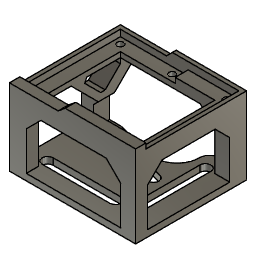
header_bus_mount v4 (Autodesk Fusion 360 design; units mm, degrees)
Autodesk Fusion 360 part; units mm, degrees
sketch "Sketch1" plane through (0, 0, 0) normal (0, 0, 1) x (1, 0, 0)
  line L0 (17.22, 32.84) -> (37.54, 32.84) construction
  line L1 (37.54, 32.84) -> (37.54, 1.4) construction
  line L2 (37.54, 1.4) -> (17.22, 1.4) construction
  line L3 (17.22, 1.4) -> (17.22, 32.84) construction
  line L4 (1.4, 32.84) -> (21.72, 32.84) construction
  line L5 (21.72, 32.84) -> (21.72, 1.4) construction
  line L6 (21.72, 1.4) -> (1.4, 1.4) construction
  line L7 (1.4, 1.4) -> (1.4, 32.84) construction
  line L8 (1.2, 33.04) -> (37.74, 33.04)
  line L9 (37.74, 33.04) -> (37.74, 1.2)
  line L10 (37.74, 1.2) -> (1.2, 1.2)
  line L11 (1.2, 1.2) -> (1.2, 33.04)
  line L12 (38.94, 34.24) -> (38.94, 0)
  line L13 (38.94, 0) -> (0, 0)
  line L14 (0, 0) -> (0, 34.24)
  line L15 (0, 34.24) -> (38.94, 34.24)
  dimension "d5" = 20.32
  dimension "d6" = 31.44
  dimension "d7" = 4.5
  dimension "d14" = 0.2
  dimension "d15" = 0.2
  dimension "d16" = 0.2
  dimension "d17" = 0.2
  constraint horizontal L0
  constraint vertical L1
  constraint horizontal L2
  constraint vertical L3
  constraint horizontal L4
  constraint vertical L5
  constraint horizontal L6
  constraint vertical L7
  constraint coincident L2 L5.end
  constraint equal L0 L4
  constraint equal L1 L7
  constraint horizontal L8
  constraint vertical L9
  constraint horizontal L10
  constraint vertical L11
  constraint coincident L13.end L14.start
  measures "d5" distance of L0.start L0.end
  measures "d6" distance of L0.end L1.end
  measures "d7" distance of L3 L5
  measures "d14" distance of L4 L8
  measures "d15" distance of L6 L10
  measures "d16" distance of L7 L11
  measures "d17" distance of L1 L9
extrude "Extrude1" add sketch "Sketch1" along normal blind 2 makes body 1
sketch "Sketch2" plane through (0, 0, 0) normal (0, 0, -1) x (1, 0, 0)
  line L0 (1.2, -1.2) -> (37.74, -1.2)
  line L1 (37.74, -1.2) -> (37.74, -33.04)
  line L2 (37.74, -33.04) -> (1.2, -33.04)
  line L3 (1.2, -33.04) -> (1.2, -1.2)
  line L4 (0, 0) -> (0, -34.24)
  line L5 (0, -34.24) -> (38.94, -34.24)
  line L6 (38.94, -34.24) -> (38.94, 0)
  line L7 (38.94, 0) -> (0, 0)
  line L8 (5.2, -3.7) -> (34.34, -3.7)
  line L9 (34.34, -3.7) -> (34.34, -29.04)
  line L10 (34.34, -29.04) -> (5.2, -29.04)
  line L11 (5.2, -29.04) -> (5.2, -3.7)
  dimension "d21" = 4
  dimension "d22" = 3.4
  dimension "d23" = 4
  dimension "d24" = 2.5
  constraint horizontal L8
  constraint vertical L9
  constraint horizontal L10
  constraint vertical L11
  measures "d21" distance of L2 L10
  measures "d22" distance of L1 L9
  measures "d23" distance of L3 L11
  measures "d24" distance of L0 L8
extrude "Extrude2" add sketch "Sketch2" along normal blind 1.6 contours L0 L1 L2 L3 | L4 L5 L6 L7 bodies 1
sketch "Sketch3" plane through (0, 0, 2) normal (0, 0, 1) x (-1, 0, 0)
  line L0 (-37.74, -1.2) -> (-1.2, -1.2)
  line L1 (-1.2, -1.2) -> (-1.2, -33.04)
  line L2 (-1.2, -33.04) -> (-37.74, -33.04)
  line L3 (-37.74, -33.04) -> (-37.74, -1.2)
  line L4 (0, -34.24) -> (0, 0)
  line L5 (0, 0) -> (-38.94, 0)
  line L6 (-38.94, 0) -> (-38.94, -34.24)
  line L7 (-38.94, -34.24) -> (0, -34.24)
  line L8 (-17.22, -1.4) -> (-17.22, -32.84) construction
  line L9 (-17.22, -34.24) -> (-17.22, -33.04)
  line L10 (-17.22, -1.2) -> (-17.22, 0)
  constraint coincident L7 L9.start
  constraint coincident L2 L9.end
  constraint perpendicular L2 L9
  constraint coincident L0 L10.start
  constraint coincident L5 L10.end
  constraint perpendicular L5 L10
  constraint collinear L8 L10
  constraint collinear L8 L9
extrude "Extrude3" add sketch "Sketch3" along normal blind 1.8 contours L0 L2 L3 L5 L6 L7 L9 L10 bodies 1
sketch "Sketch4" plane through (0, 0, 0) normal (0, 0, 1) x (-1, 0, 0)
  line L0 (-5.2, -29.04) -> (-34.34, -29.04)
  line L1 (-34.34, -29.04) -> (-34.34, -3.7)
  line L2 (-34.34, -3.7) -> (-5.2, -3.7)
  line L3 (-5.2, -3.7) -> (-5.2, -29.04)
  line L4 (-37.74, -1.2) -> (-37.74, -33.04)
  line L5 (-37.74, -33.04) -> (-1.2, -33.04)
  line L6 (-1.2, -33.04) -> (-1.2, -1.2)
  line L7 (-1.2, -1.2) -> (-37.74, -1.2)
  line L8 (-21.72, -32.84) -> (-21.72, -1.4) construction
  line L9 (-22.12, -1.2) -> (-22.12, -33.04)
  dimension "d29" = 0.4
  constraint coincident L7 L9.start
  constraint coincident L5 L9.end
  constraint perpendicular L5 L9
  measures "d29" distance of L8 L9
extrude "Extrude4" add sketch "Sketch4" along normal blind 1.6 contours L0 L1 L2 L4 L5 L7 L9 bodies 1
sketch "Sketch5" plane through (0, 0, 0) normal (0, 0, 1) x (-1, 0, 0)
  line L0 (-22.12, -29.04) -> (-22.12, -33.04)
  line L1 (-22.12, -33.04) -> (-1.2, -33.04)
  line L2 (-1.2, -33.04) -> (-1.2, -1.2)
  line L3 (-1.2, -1.2) -> (-22.12, -1.2)
  line L4 (-22.12, -1.2) -> (-22.12, -3.7)
  line L5 (-22.12, -3.7) -> (-5.2, -3.7)
  line L6 (-5.2, -3.7) -> (-5.2, -29.04)
  line L7 (-5.2, -29.04) -> (-22.12, -29.04)
  circle A0 centre (-3.2, -31.04) radius 1
  circle A1 centre (-19.2, -31.04) radius 1
  circle A2 centre (-35.94, -31.04) radius 1
  line L8 (-1.2, -1.2) -> (-1.2, -33.04)
  line L9 (-1.2, -33.04) -> (-17.22, -33.04)
  line L10 (-37.74, -33.04) -> (-37.74, -1.2) construction
  dimension "d33" = 2
  dimension "d34" = 2
  dimension "d35" = 1.8
  dimension "d36" = 18
  dimension "d37" = 2
  constraint horizontal A0.centre A1.centre
  constraint horizontal A1.centre A2.centre
  constraint equal A0 A1
  constraint equal A1 A2
  measures "d33" distance of A0.centre L8
  measures "d34" distance of A0.centre L9
  measures "d35" distance of A2.centre L10
  measures "d36" distance of A1.centre L8
  measures "d37" diameter of A0
extrude "Extrude5" cut sketch "Sketch5" along normal up to surface (-1.6 mm away) and the other way up to surface (-1.6 mm away) contours A0 | A1 | A2 bodies 1
sketch "Sketch6" plane through (0, 0, 2) normal (0, 0, 1) x (-1, 0, 0)
  line L0 (-17.22, -33.04) -> (-17.22, -34.24)
  line L1 (-17.22, -34.24) -> (0, -34.24)
  line L2 (0, -34.24) -> (0, 0)
  line L3 (0, 0) -> (-17.22, 0)
  line L4 (-17.22, 0) -> (-17.22, -1.2)
  line L5 (-17.22, -1.2) -> (-1.2, -1.2)
  line L6 (-1.2, -1.2) -> (-1.2, -33.04)
  line L7 (-1.2, -33.04) -> (-17.22, -33.04)
  line L8 (0, 0) -> (0, -3.2)
  line L9 (0, -3.2) -> (-17.02, -3.2)
  line L10 (-17.02, -3.2) -> (-17.02, 0)
  line L11 (0, 0) -> (-17.02, 0)
  line L12 (-17.22, -1.2) -> (-17.22, 0)
  dimension "d47" = 0.2
  dimension "d48" = 3.2
  constraint vertical L8
  constraint horizontal L9
  constraint coincident L2 L8.end
  constraint coincident L3 L10.end
  constraint perpendicular L3 L10
  constraint perpendicular L10 L11
  measures "d47" distance of L10 L12
  measures "d48" distance of L9 L11
extrude "Extrude6" add sketch "Sketch6" along normal blind 1.6 contours L5 L6 L9 L10 | L2 L3 L5 L6 L8 L9 L10 L11 | L3 L4 L5 L10 L12 bodies 1
sketch "Sketch7" plane through (0, 0, 3.8) normal (0, 0, 1) x (-1, 0, 0)
  line L0 (-17.22, -1.2) -> (-17.22, 0)
  line L1 (-17.22, 0) -> (-38.94, 0)
  line L2 (-38.94, 0) -> (-38.94, -34.24)
  line L3 (-38.94, -34.24) -> (-17.22, -34.24)
  line L4 (-17.22, -34.24) -> (-17.22, -33.04)
  line L5 (-17.22, -33.04) -> (-37.74, -33.04)
  line L6 (-37.74, -33.04) -> (-37.74, -1.2)
  line L7 (-37.74, -1.2) -> (-17.22, -1.2)
  line L8 (-38.94, 0) -> (-17.22, 0)
  line L9 (-17.22, 0) -> (-17.22, -3.2)
  line L10 (-17.22, -3.2) -> (-38.94, -3.2)
  line L11 (-38.94, -3.2) -> (-38.94, 0)
  line L12 (-17.02, -3.2) -> (0, -3.2)
  point P0 (-17.02, -3.2)
  point P1 (0, -3.2)
  constraint horizontal L8
  constraint vertical L9
  constraint horizontal L10
  constraint vertical L11
  constraint coincident L1.end L2.start
  constraint coincident L0.end L1.start
  constraint collinear L10 L12
extrude "Extrude7" add sketch "Sketch7" along normal blind 1.6 contours L0 L1 L2 L6 L7 L8 L9 L10 L11 | L6 L7 L9 L10 bodies 1
sketch "Sketch8" plane through (0, 3.2, 0) normal (0, 1, 0) x (-1, 0, 0)
  line L0 (-37.74, 3.8) -> (-17.22, 3.8)
  line L1 (-17.22, 3.8) -> (-17.22, 5.4)
  line L2 (-17.22, 5.4) -> (-38.94, 5.4)
  line L3 (-38.94, 5.4) -> (-38.94, 3.8)
  line L4 (-38.94, 3.8) -> (-37.74, 3.8)
  line L5 (-17.22, 5.4) -> (-15.02, 3.6)
  line L6 (-15.02, 3.6) -> (-17.02, 3.6)
  line L7 (-17.02, 3.6) -> (-17.02, 3.8)
  line L8 (-17.02, 3.8) -> (-17.22, 3.8)
  line L9 (-17.22, 3.8) -> (-17.22, 5.4)
  point P0 (-17.02, 3.6)
  dimension "d49" = 2
  constraint coincident L1.end L2.start
  constraint perpendicular L1 L6
  constraint perpendicular L0 L7
  constraint coincident L0.end L1.start
  constraint perpendicular L1 L8
  constraint coincident P0 L6.end
  measures "d49" distance of L5.end P0
extrude "Extrude8" add sketch "Sketch8" against normal up to surface (3.2 mm away) contours L1 L5 L6 L7 L8 L9 bodies 1
chamfer "Chamfer1" distance 1.8 angle 45 1 edges at (17.22, 33.64, 2) on bodies 1
sketch "Sketch9" plane through (0, 0, 0) normal (0, -1, 0) x (1, 0, 0)
  line L0 (17.22, 3.8) -> (17.22, 3.6)
  line L1 (17.22, 3.6) -> (17.02, 3.6)
  line L2 (17.02, 3.6) -> (17.02, 3.8)
  line L3 (17.02, 3.8) -> (17.22, 3.8)
  line L4 (17.22, 5.4) -> (15.02, 3.6)
  line L5 (15.02, 3.6) -> (0, 3.6)
  line L6 (0, 3.6) -> (0, -1.6)
  line L7 (0, -1.6) -> (38.94, -1.6)
  line L8 (38.94, -1.6) -> (38.94, 5.4)
  line L9 (38.94, 5.4) -> (17.22, 5.4)
extrude "Extrude9" add sketch "Sketch9" against normal up to surface (1.2 mm away) contours L0 L1 L2 L3 bodies 1
ref_plane "WorkPlane1" through (0, 0, -20) normal (0, 0, 1) x (1, 0, 0)
sketch "Sketch11" plane through (0, 0, -20) normal (0, 0, 1) x (1, 0, 0)
  line L0 (38.94, 0) -> (0, 0)
  line L1 (38.94, 34.24) -> (38.94, 0)
  line L2 (0, 34.24) -> (38.94, 34.24)
  line L3 (0, 0) -> (0, 34.24)
  line L4 (5.2, 29.04) -> (5.2, 3.7) construction
  line L5 (5.2, 3.7) -> (34.34, 3.7) construction
  line L6 (34.34, 3.7) -> (34.34, 29.04) construction
  line L7 (34.34, 29.04) -> (5.2, 29.04) construction
  circle A0 centre (3.2, 31.04) radius 1 construction
  circle A1 centre (19.2, 31.04) radius 1 construction
  circle A2 centre (35.94, 31.04) radius 1 construction
  line L8 (0, 27.24) -> (23, 27.24)
  line L9 (23, 27.24) -> (23, 34.24)
  line L10 (5.2, 4.9) -> (26.04, 4.9)
  arc A3 (26.04, 4.9) -> (26.04, 8.3) centre (26.04, 6.6) ccw
  line L11 (26.04, 8.3) -> (5.2, 8.3)
  arc A4 (5.2, 8.3) -> (5.2, 4.9) centre (5.2, 6.6) ccw
  line L12 (29.74, 29.04) -> (29.74, 6.6)
  arc A5 (29.74, 6.6) -> (33.14, 6.6) centre (31.44, 6.6) ccw
  line L13 (33.14, 6.6) -> (33.14, 29.04)
  arc A6 (33.14, 29.04) -> (29.74, 29.04) centre (31.44, 29.04) ccw
  line L14 (31.44, 29.04) -> (31.44, 6.6) construction
  line L15 (26.04, 6.6) -> (5.2, 6.6) construction
  line L16 (26.04, 6.6) -> (27.74, 6.6) construction
  line L17 (29.74, 6.6) -> (31.44, 6.6) construction
  line L18 (27.74, 6.6) -> (29.74, 6.6) construction
  line L19 (6.46, 21.8979) -> (25.6, 16.7694)
  arc A7 (25.6, 16.7694) -> (26.48, 20.0535) centre (26.04, 18.4115) ccw
  line L20 (26.48, 20.0535) -> (7.34, 25.1821)
  arc A8 (7.34, 25.1821) -> (6.46, 21.8979) centre (6.9, 23.54) ccw
  line L21 (6.9, 23.54) -> (26.04, 18.4115) construction
  line L22 (27.74, 15.5565) -> (27.74, 24.5386) construction
  line L23 (2.9112, 25.24) -> (12.3922, 25.24) construction
  line L24 (7.3871, 27.24) -> (27.74, 21.7865)
  line L25 (27.74, 21.7865) -> (27.74, 34.24)
  point P0 (3.5, 6.6)
  point P1 (27.74, 6.6)
  point P2 (31.44, 4.9)
  point P3 (31.44, 30.74)
  dimension "d57" = 23
  dimension "d58" = 7
  dimension "d60" = 1.7
  dimension "d62" = 1.2
  dimension "d63" = 1.2
  dimension "d64" = 2
  dimension "d65" = 2
  dimension "d66" = 2
  dimension "d67" = 15
  dimension "d68" = 2
  constraint coincident L3 L8.start
  constraint perpendicular L3 L8
  constraint coincident L2 L9.end
  constraint perpendicular L2 L9
  constraint tangent L10 A3
  constraint tangent A3 L11
  constraint parallel L10 L11
  constraint tangent L11 A4
  constraint tangent L10 A4
  constraint tangent L12 A5
  constraint tangent A5 L13
  constraint parallel L12 L13
  constraint tangent L13 A6
  constraint tangent L12 A6
  constraint parallel L6 L14
  constraint equal A3 A5
  constraint midpoint A4 P0
  constraint midpoint A3 P1
  constraint midpoint A5 P2
  constraint midpoint A6 P3
  constraint coincident A3.centre L15.start
  constraint coincident A4.centre L15.end
  constraint horizontal L15
  constraint coincident L4 A4.centre
  constraint coincident L7 A6.centre
  constraint coincident A3 P1
  constraint coincident A5 L12.end
  constraint coincident A5.centre L14.end
  constraint parallel L16 L18
  constraint parallel L17 L18
  constraint horizontal L17
  constraint tangent L19 A7
  constraint tangent A7 L20
  constraint parallel L19 L20
  constraint tangent L20 A8
  constraint tangent L19 A8
  constraint equal A3 A7
  constraint vertical L22
  constraint tangent A7 L22
  constraint perpendicular L4 L23
  constraint tangent A8 L23
  constraint coincident L8 L24.start
  constraint coincident L2 L25.end
  constraint perpendicular L2 L25
  constraint parallel L21 L24
  constraint coincident L22.end L25
  constraint tangent L4 A8
  measures "d57" distance of L8.start L8.end
  measures "d58" distance of L8.end L9.end
  measures "d60" radius of A4
  measures "d62" distance of L5 L10
  measures "d63" distance of L6 L13
  measures "d64" distance of P1 L12.end
  measures "d65" distance of L12 L22
  measures "d66" distance of L8 L23
  measures "d67" angle of L21 L23
  measures "d68" distance of L20 L24
extrude "Extrude10" add sketch "Sketch11" along normal blind 2 separate body contours L0 L1 L2 L3 L8 L24 L25 makes body 2
fillet "Fillet1" radius 7 1 edges at (27.74, 21.7865, -19) on bodies 2
fillet "Fillet1" radius 7 1 edges at (7.3871, 27.24, -19) on bodies 2
sketch "Sketch12" plane through (0, 0, -1.6) normal (0, 0, -1) x (1, 0, 0)
  circle A0 centre (3.2, -31.04) radius 1
  circle A1 centre (19.2, -31.04) radius 1
  circle A2 centre (35.94, -31.04) radius 1
  line L0 (34.34, -29.04) -> (5.2, -29.04)
  line L1 (5.2, -29.04) -> (5.2, -3.7)
  line L2 (5.2, -3.7) -> (34.34, -3.7)
  line L3 (34.34, -3.7) -> (34.34, -29.04)
  line L4 (38.94, 0) -> (0, 0)
  line L5 (0, 0) -> (0, -34.24)
  line L6 (0, -34.24) -> (38.94, -34.24)
  line L7 (38.94, -34.24) -> (38.94, 0)
  line L8 (5.2, -3.7) -> (0, -3.7)
  line L9 (0, -3.7) -> (0, 0)
  line L10 (0, 0) -> (5.2, 0)
  line L11 (5.2, 0) -> (5.2, -3.7)
  line L12 (5.2, -29.04) -> (0, -29.04)
  line L13 (0, -29.04) -> (0, -34.24)
  line L14 (0, -34.24) -> (5.2, -34.24)
  line L15 (5.2, -34.24) -> (5.2, -29.04)
  line L16 (34.34, -29.04) -> (38.94, -29.04)
  line L17 (38.94, -29.04) -> (38.94, -34.24)
  line L18 (38.94, -34.24) -> (34.34, -34.24)
  line L19 (34.34, -34.24) -> (34.34, -29.04)
  line L20 (34.34, -3.7) -> (38.94, -3.7)
  line L21 (38.94, -3.7) -> (38.94, 0)
  line L22 (38.94, 0) -> (34.34, 0)
  line L23 (34.34, 0) -> (34.34, -3.7)
  constraint horizontal L8
  constraint vertical L9
  constraint horizontal L10
  constraint vertical L11
  constraint coincident L4.end L5.start
  constraint coincident L1.end L2.start
  constraint horizontal L12
  constraint vertical L13
  constraint horizontal L14
  constraint vertical L15
  constraint coincident L5.end L6.start
  constraint coincident L0.end L1.start
  constraint horizontal L16
  constraint vertical L17
  constraint horizontal L18
  constraint vertical L19
  constraint coincident L6.end L7.start
  constraint coincident L0.start L3.end
  constraint horizontal L20
  constraint vertical L21
  constraint horizontal L22
  constraint vertical L23
  constraint coincident L4.start L7.end
  constraint coincident L2.end L3.start
extrude "Extrude11" add sketch "Sketch12" along normal up to surface (8.4 mm away) contours L5 L6 L12 L13 L14 L15 bodies 1
extrude "Extrude12" add sketch "Sketch12" along normal up to surface (16.4 mm away) contours L6 L7 L16 L17 L18 L19 | L4 L7 L20 L21 L22 L23 | L4 L5 L8 L9 L10 L11 bodies 1 2
sketch "Sketch13" plane through (0, 0, -18) normal (0, 0, 1) x (-1, 0, 0)
  line L0 (-5.2, -3.7) -> (-5.2, 0)
  line L1 (-5.2, 0) -> (-34.34, 0)
  line L2 (-34.34, 0) -> (-34.34, -3.7)
  line L3 (-34.34, -3.7) -> (-38.94, -3.7)
  line L4 (-38.94, -3.7) -> (-38.94, -29.04)
  line L5 (-38.94, -29.04) -> (-34.34, -29.04)
  line L6 (-34.34, -29.04) -> (-34.34, -34.24)
  line L7 (-34.34, -34.24) -> (-27.74, -34.24)
  line L8 (-27.74, -34.24) -> (-27.74, -30.909)
  arc A0 (-18.9283, -24.1476) -> (-27.74, -30.909) centre (-20.74, -30.909) ccw
  line L9 (-18.9283, -24.1476) -> (-8.2773, -27.0015)
  arc A1 (-8.2773, -27.0015) -> (-6.4655, -27.24) centre (-6.4655, -20.24) ccw
  line L10 (-6.4655, -27.24) -> (0, -27.24)
  line L11 (0, -27.24) -> (0, -3.7)
  line L12 (0, -3.7) -> (-5.2, -3.7)
  arc A2 (-5.2, -8.3) -> (-5.2, -4.9) centre (-5.2, -6.6) ccw
  line L13 (-5.2, -8.3) -> (-26.04, -8.3)
  arc A3 (-26.04, -4.9) -> (-26.04, -8.3) centre (-26.04, -6.6) ccw
  line L14 (-26.04, -4.9) -> (-5.2, -4.9)
  arc A4 (-7.34, -25.1821) -> (-6.46, -21.8979) centre (-6.9, -23.54) ccw
  line L15 (-7.34, -25.1821) -> (-26.48, -20.0535)
  arc A5 (-25.6, -16.7694) -> (-26.48, -20.0535) centre (-26.04, -18.4115) ccw
  line L16 (-25.6, -16.7694) -> (-6.46, -21.8979)
  arc A6 (-33.14, -29.04) -> (-29.74, -29.04) centre (-31.44, -29.04) ccw
  line L17 (-33.14, -29.04) -> (-33.14, -6.6)
  arc A7 (-29.74, -6.6) -> (-33.14, -6.6) centre (-31.44, -6.6) ccw
  line L18 (-29.74, -6.6) -> (-29.74, -29.04)
  line L19 (0, -27.24) -> (-3.7, -27.24)
  line L20 (-3.7, -27.24) -> (-3.7, -22.24)
  line L21 (-3.7, -22.24) -> (0, -22.24)
  line L22 (0, -22.24) -> (0, -27.24)
  line L23 (-6.9, -23.54) -> (-5.2, -23.54) construction
  dimension "d79" = 1.5
  dimension "d80" = 5
  constraint horizontal L19
  constraint vertical L20
  constraint horizontal L21
  constraint vertical L22
  constraint coincident L10.end L11.start
  constraint coincident A4.centre L23.start
  constraint coincident A4 L23.end
  constraint horizontal L23
  measures "d79" distance of L20 L23.end
  measures "d80" distance of L10.end L21.end
extrude "Extrude13" add sketch "Sketch13" along normal up to surface (8 mm away) contours L10 L11 L19 L20 L21 L22 bodies 1
sketch "Sketch14" plane through (0, 0, 0) normal (-1, 0, 0) x (0, -1, 0)
  line L0 (-27.24, -20) -> (0, -20)
  line L1 (0, -20) -> (0, 3.6)
  line L2 (0, 3.6) -> (-3.2, 3.6)
  line L3 (-3.2, 3.6) -> (-3.2, 2)
  line L4 (-3.2, 2) -> (-34.24, 2)
  line L5 (-34.24, 2) -> (-34.24, -10)
  line L6 (-34.24, -10) -> (-29.04, -10)
  line L7 (-29.04, -10) -> (-29.04, -1.6)
  line L8 (-29.04, -1.6) -> (-3.7, -1.6)
  line L9 (-3.7, -1.6) -> (-3.7, -18)
  line L10 (-3.7, -18) -> (-22.24, -18)
  line L11 (-22.24, -18) -> (-22.24, -10)
  line L12 (-22.24, -10) -> (-27.24, -10)
  line L13 (-27.24, -10) -> (-27.24, -20)
  line L14 (-27.24, -10) -> (-29.04, -10)
  line L15 (-29.04, -10) -> (-29.04, -3.2)
  line L16 (-29.04, -3.2) -> (-22.24, -10)
  line L17 (-27.24, -10) -> (-22.24, -10)
  dimension "d83" = 45
  constraint coincident L12.end L13.start
  constraint coincident L6.end L7.start
  constraint coincident L7 L15.end
  constraint perpendicular L6 L15
  constraint coincident L11.end L12.start
  measures "d83" angle of L16 L17
extrude "Extrude14" add sketch "Sketch14" against normal up to surface (5.2 mm away) contours L7 L12 L14 L15 L16 L17 bodies 1
chamfer "Chamfer2" distance 1.5 angle 45 1 edges at (3.7, 24.74, -10) on bodies 1
chamfer "Chamfer3" distance 7 angle 45 1 edges at (2.6, 34.24, -10) on bodies 1
chamfer "Chamfer4" distance 4.5 angle 45 6 edges at (5.2, 1.85, -1.6) (34.34, 1.85, -1.6) (36.64, 3.7, -1.6) (36.64, 29.04, -1.6) (34.34, 31.64, -1.6) (2.6, 3.7, -1.6) on bodies 1
sketch "Sketch15" plane through (0, 0, 0) normal (-1, 0, 0) x (0, -1, 0)
  line L0 (-22.24, -10) -> (-29.04, -3.2)
  line L1 (-29.04, -3.2) -> (-29.04, -1.6)
  line L2 (-29.04, -1.6) -> (-8.2, -1.6)
  line L3 (-8.2, -1.6) -> (-3.7, -6.1)
  line L4 (-3.7, -6.1) -> (-3.7, -18)
  line L5 (-3.7, -18) -> (-22.24, -18)
  line L6 (-22.24, -18) -> (-22.24, -10)
  line L7 (-34.24, -3) -> (-27.24, -10)
  line L8 (-27.24, -10) -> (-27.24, -20)
  line L9 (-27.24, -20) -> (0, -20)
  line L10 (0, -20) -> (0, 3.6)
  line L11 (0, 3.6) -> (-3.2, 3.6)
  line L12 (-3.2, 3.6) -> (-3.2, 2)
  line L13 (-3.2, 2) -> (-34.24, 2)
  line L14 (-34.24, 2) -> (-34.24, -3)
  line L15 (-22.24, -10) -> (-13.84, -1.6)
  line L16 (-23.6542, -8.5858) -> (-16.6684, -1.6)
  line L17 (-23.6542, -8.5858) -> (-22.24, -10)
  line L18 (-16.6684, -1.6) -> (-13.84, -1.6)
  dimension "d90" = 45
  dimension "d91" = 2
  constraint coincident L0.start L6.end
  constraint coincident L2 L15.end
  constraint coincident L0 L16.start
  constraint coincident L2 L16.end
  constraint parallel L15 L16
  measures "d90" angle of L2 L15
  measures "d91" distance of L15 L16
extrude "Extrude15" add sketch "Sketch15" against normal up to surface (5.1997 mm away) contours L0 L2 L15 L16 L17 L18 bodies 1
chamfer "Chamfer5" distance 2 angle 45 1 edges at (2.6, 16.6684, -1.6) on bodies 1
chamfer "Chamfer6" distance 1 angle 45 1 edges at (2.6, 23.6542, -8.5858) on bodies 1
fillet "Fillet2" radius 3.5 1 edges at (27.74, 34.24, -19) on bodies 1
equation "perf_L = 31.44 mm"
equation "perf_W = 20.32 mm"
equation "perf_t = 1.6 mm"
equation "perf_overlap = 4.5 mm"
equation "d5 = perf_W"
equation "d6 = perf_L"
equation "d7 = perf_overlap"
equation "wall_t = 1.2 mm"
equation "floor_t = 1.6 mm"
equation "clearance = 0.2 mm"
equation "d14 = clearance"
equation "d15 = clearance"
equation "d16 = clearance"
equation "d17 = clearance"
equation "d18 = -wall_t"
equation "d19 = perf_t + clearance * 2"
equation "d25 = floor_t"
equation "d27 = perf_t + clearance"
equation "d29 = clearance * 2"
equation "d30 = perf_t"
equation "M2_D = 2 mm"
equation "d37 = M2_D"
equation "d43 = floor_t"
equation "d45 = floor_t"
equation "d47 = clearance"
equation "standoff_H = 20 mm"
equation "d56 = -standoff_H"
equation "M3_D = 3 mm"
equation "d60 = M3_D / 2 + clearance"
